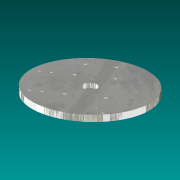
# Autodesk Inventor part: base bovenkant v2
Saved by Autodesk Inventor 2020.3 (Build 243373000, 373)
## iProperties
Created: 2020-05-15
Part Number: base bovenkant v2
Material: Aluminum 6061
Document SubType Name: Modeling
Designer: Svend
Density: 2.7 g/cm^3
Appearance: Aluminum - Polished
Author: Svend
Autodesk Inventor part; units mm, degrees
ref_plane "YZ Plane" through (0, 0, 0) normal (1, 0, 0) x (0, 1, 0)
ref_plane "XZ Plane" through (0, 0, 0) normal (0, 1, 0) x (-1, 0, 0)
ref_plane "XY Plane" through (0, 0, 0) normal (0, 0, 1) x (1, 0, 0)
sketch "Sketch1" plane through (0, 0, 0) normal (0, 0, 1) x (1, 0, 0)
  circle A0 centre (-11.3135, -11.3135) radius 2
  circle A1 centre (-11.3135, 11.3135) radius 2
  circle A2 centre (11.3135, 11.3135) radius 2
  circle A3 centre (11.3135, -11.3135) radius 2
  circle A4 centre (-15.3135, 11.3135) radius 2
  circle A5 centre (-7.3135, 11.3135) radius 2
  circle A6 centre (7.3135, 11.3135) radius 2
  circle A7 centre (15.3135, 11.3135) radius 2
  circle A8 centre (15.3135, -11.3135) radius 2
  circle A9 centre (7.3135, -11.3135) radius 2
  circle A10 centre (-7.3135, -11.3135) radius 2
  circle A11 centre (-15.3135, -11.3135) radius 2
  line L0 (-15.3135, 13.3135) -> (-7.3135, 13.3135)
  line L1 (-7.3135, 9.3135) -> (-15.3135, 9.3135)
  line L2 (-15.3135, -9.3135) -> (-7.3135, -9.3135)
  line L3 (-7.3135, -13.3135) -> (-15.3135, -13.3135)
  line L4 (7.3135, -9.3135) -> (15.3135, -9.3135)
  line L5 (15.3135, -13.3135) -> (7.3135, -13.3135)
  line L6 (15.3135, 9.3135) -> (7.3135, 9.3135)
  line L7 (15.3135, 13.3135) -> (7.3135, 13.3135)
  circle A12 centre (0, 0) radius 8.25
  circle A13 centre (5, 0) radius 8.25
  circle A14 centre (-5, 0) radius 8.25
  line L8 (-5, 8.25) -> (5, 8.25)
  line L9 (5, -8.25) -> (-5, -8.25)
  circle A15 centre (0, 0) radius 42.5
  circle A16 centre (59.509, 0) radius 50.7821
  line L10 (-5.9149, 42.0864) -> (52.4415, 50.2878)
  line L11 (-5.9149, -42.0864) -> (52.4415, -50.2878)
  line L12 (-13.25, 0) -> (13.25, 0)
  circle A17 centre (59.509, 0) radius 11
  arc A18 (-5.9149, 42.0864) -> (-5.9149, -42.0864) centre (0, 0) ccw
  line L13 (-42.5, 0) -> (156.5802, 0)
  circle A19 centre (59.509, 0) radius 90
  point P0 (-3.1314, -32.3793)
  point P1 (23.2633, -35.5678)
  point P2 (23.2633, 35.5678)
  point P3 (-2.5, -7.8621)
  point P4 (0, -8.25)
  dimension "d0" = 4
  dimension "d1" = 22.627
  dimension "d2" = 22.627
  dimension "d3" = 11.3135
  dimension "d4" = 11.3135
  dimension "d5" = 4
  dimension "d6" = 4
  dimension "d7" = 4
  dimension "d8" = 4
  dimension "d9" = 4
  dimension "d10" = 4
  dimension "d11" = 4
  dimension "d12" = 4
  dimension "d15" = 16.5
  dimension "d16" = 5
  dimension "d17" = 5
  dimension "d18" = 85
  dimension "d19" = 8
  dimension "d20" = 59.509
  dimension "d21" = 22
  dimension "d24" = 85
  dimension "d116" = 180
  constraints: 29 point on circle, 28 end point, 20 centre point, 13 equal radius, 13 horizontal alignment, 10 tangent, 9 point on line, 5 coincident, 4 parallel, 3 horizontal, 2 midpoint, 2 vertical alignment
  measures "d0" diameter of A0
  measures "d1" distance of A1.centre A2.centre
  measures "d2" distance of A3.centre A2.centre
  measures "d3" horizontal distance of point (0, 0) A1.centre
  measures "d4" horizontal distance of point (0, 0) A1.centre
  measures "d5" distance of A2.centre A6.centre
  measures "d6" distance of A7.centre A2.centre
  measures "d7" distance of A3.centre A8.centre
  measures "d8" distance of A9.centre A3.centre
  measures "d9" distance of A0.centre A10.centre
  measures "d10" distance of A11.centre A0.centre
  measures "d11" distance of A1.centre A4.centre
  measures "d12" distance of A5.centre A1.centre
  measures "d15" diameter of A12
  measures "d16" distance of A14.centre A12.centre
  measures "d17" distance of A12.centre A13.centre
  measures "d18" diameter of A15
  measures "d19" angle of L12 L10
  measures "d20" distance of A16.centre point (0, 0)
  measures "d21" diameter of A17
  measures "d24" diameter of A18
  measures "d116" diameter of A19
extrude "Extrusion1" add sketch "Sketch1" along normal blind 10 contours A0 | A10 L3 A0 | A0 L2 A10 | A10 | A0 A11 L2 | L3 A11 A0 | A11 | A1 | A5 L1 A1 | A1 L0 A5 | A5 | A1 A4 L0 | L1 A4 A1 | A4 | A2 A16 | A7 L6 A2 | A2 L7 A7 | A7 | L7 A16 A15 L13 A13 L6 A7 | A2 A16 L7 | L6 A16 A2 | A16 A2 | A2 A6 L7 A16 | L7 A6 L6 A16 A13 L8 A14 L13 A19 A15 | A16 L6 A6 A2 | A6 | A16 L13 A17 A15 | A15 L10 A16 | A16 L12 A12 A13 | A13 L12 A16 | L13 A17 A16 A15 | A15 A16 L5 A8 L4 A13 L13 | A15 A19 L13 A16 L10 | A13 A16 L12 | A13 A12 L8 | A16 A13 A12 L12 | A16 L11 A15 | A15 A19 L13 A14 L9 A13 A16 L4 A9 L5 | L13 A19 A15 L11 A16 | A13 A14 A12 | A12 L12 A14 A13 | A12 A14 L8 | A12 A13 A14 L12 | A16 A3 L5 | L5 A9 A3 A16 | L9 A12 A13 | A16 A3 A9 L4 | L4 A3 A16 | A14 L12 A13 | A13 L12 A12 A14 | A12 L12 A14 | A12 A14 A13 | A14 A13 L12 | A3 A16 | A3 A8 L5 | A9 | A3 A16 | L12 A12 A14 | L9 A14 A12 | L4 A8 A3 | A13 A14 A12 L12 | A8
sketch "Sketch18" plane through (59.509, 0, 0) normal (0, 0, -1) x (-1, 0, 0)
  circle A0 centre (0, 0) radius 35
  circle A1 centre (0, 0) radius 90 projected
  circle A2 centre (0, 0) radius 11 projected
  circle A3 centre (0, 0) radius 16
  point P0 (59.509, 0)
  dimension "d127" = 70
  dimension "d130" = 5
  constraints: 2 centre point, 1 coincident
  measures "d127" diameter of A0
  measures "d130" radial gap between concentric circles of A2 A3
extrude "Extrusion9" cut sketch "Sketch18" against normal blind 6.5 contours A0 | A2
sketch "Sketch20" plane through (59.509, 0, 0) normal (0, 0, -1) x (-1, 0, 0)
  circle A0 centre (0, 0) radius 11 projected
  circle A1 centre (0, 0) radius 11 projected
  circle A2 centre (0, 0) radius 6
  point P0 (59.509, 0)
  dimension "d136" = 12
  constraints: 1 centre point, 1 coincident
  measures "d136" diameter of A2
extrude "Extrusion11" add sketch "Sketch20" against normal blind 3
sketch "Sketch22" plane through (59.509, 0, 0) normal (0, 0, -1) x (-1, 0, 0)
  circle A0 centre (55.7915, 31.25) radius 1.621 projected
  circle A1 centre (71.5915, 31.25) radius 1.621 projected
  circle A2 centre (71.5915, -31.2504) radius 1.621 projected
  circle A3 centre (55.7915, -31.2504) radius 1.621 projected
  circle A4 centre (71.5915, -31.2504) radius 1.621 projected
  circle A5 centre (55.7915, -31.2504) radius 1.621 projected
  circle A6 centre (71.5915, 31.25) radius 1.621 projected
  circle A7 centre (55.7915, 31.25) radius 1.621 projected
  point P0 (59.509, 0)
hole "Hole4" at (-12.0825, 31.25, 0) at (3.7175, 31.25, 0) at (-12.0825, -31.2504, 0) at (3.7175, -31.2504, 0) direction (0, 0, 1) diameter 4.2 end through all countersink diameter 9.4 countersink angle 90 clearance for "Countersunk Flat Head Screw ISO 2009/7046" size "M4" standard "ISO"
sketch "Sketch23" plane through (59.509, 0, 0) normal (0, 0, -1) x (-1, 0, 0)
  circle A0 centre (-26.526, -31.25) radius 2.4585 projected
  circle A1 centre (26.526, -31.25) radius 2.4585 projected
  circle A2 centre (-26.526, 31.25) radius 1.621 projected
  circle A3 centre (26.526, 31.25) radius 1.621 projected
  circle A4 centre (26.526, -31.25) radius 2.4585 projected
  circle A5 centre (26.526, 31.25) radius 1.621 projected
  circle A6 centre (-26.526, -31.25) radius 2.4585 projected
  circle A7 centre (0, 0) radius 90 projected
  circle A8 centre (0, 0) radius 11 projected
  circle A9 centre (-26.526, 31.25) radius 1.621 projected
  point P0 (59.509, 0)
hole "Hole5" at (86.035, 31.25, 0) at (86.035, -31.25, 0) at (32.983, -31.25, 0) at (32.983, 31.25, 0) direction (0, 0, 1) diameter 4.5 depth 14.2 tip angle 118 countersink diameter 9.4 countersink angle 90 clearance for "Countersunk Flat Head Screw ISO 2009/7046" size "M4" standard "ISO"
sketch "Sketch24" plane through (59.509, 0, 0) normal (0, 0, -1) x (-1, 0, 0)
  circle A0 centre (-19.96, 67.25) radius 1.621 projected
  circle A1 centre (19.96, 67.25) radius 1.621 projected
  circle A2 centre (-19.96, 67.25) radius 2.1
  circle A3 centre (19.96, 67.25) radius 2.1
  point P0 (59.509, 0)
  dimension "d152" = 4.2
  dimension "d153" = 4.2
  constraints: 2 centre point, 2 coincident
  measures "d152" diameter of A2
  measures "d153" diameter of A3
hole "Hole6" at (79.469, 67.25, 0) at (39.549, 67.25, 0) direction (0, 0, 1) diameter 4.5 depth 15 tip angle 118 countersink diameter 9.4 countersink angle 90 clearance for "Countersunk Flat Head Screw ISO 2009/7046" size "M4" standard "ISO"
equation "\"d2\" = d1"
equation "\"d3\" = 0.5 * d2"
equation "\"d4\" = 0.5 * d1"
equation "\"d5\" = d0"
equation "\"d6\" = d5"
equation "\"d7\" = d6"
equation "\"d8\" = d7"
equation "\"d9\" = d5"
equation "\"d10\" = d9"
equation "\"d11\" = d10"
equation "\"d12\" = d11"
equation "\"d17\" = d16"
body "Solid1"
